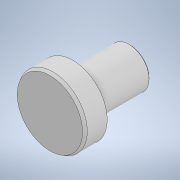
# Autodesk Inventor part: Totmannknopf
Saved by Autodesk Inventor 2021 (Build 250183000, 183)
## iProperties
Created: 2021-07-19
Part Number: Totmannknopf
Material: Generisch
Document SubType Name: Modeling
Designer: Lars-Ole
Density: 1 g/cm^3
Appearance: Vorgabe
Author: Lars-Ole
Autodesk Inventor part; units mm, degrees
ref_plane "YZ Plane" through (0, 0, 0) normal (1, 0, 0) x (0, 1, 0)
ref_plane "XZ Plane" through (0, 0, 0) normal (0, 1, 0) x (-1, 0, 0)
ref_plane "XY Plane" through (0, 0, 0) normal (0, 0, 1) x (1, 0, 0)
sketch "Skizze1" plane through (0, 0, 0) normal (0, 0, 1) x (1, 0, 0)
  line L0 (-2.05, 0.55) -> (2.05, 0.55)
  line L1 (2.05, 0.55) -> (2.05, -0.55)
  line L2 (2.05, -0.55) -> (-2.05, -0.55)
  line L3 (-2.05, -0.55) -> (-2.05, 0.55)
  line L4 (-0.65, 2.05) -> (0.65, 2.05)
  line L5 (0.65, 2.05) -> (0.65, -2.05)
  line L6 (0.65, -2.05) -> (-0.65, -2.05)
  line L7 (-0.65, -2.05) -> (-0.65, 2.05)
  circle A0 centre (0, 0) radius 3.5
  line L8 (-4.9, 0) -> (4.9, 0) construction
  line L9 (0, -4.9) -> (0, 4.9) construction
  point P0 (0.65, -0.55)
  point P1 (-0.65, -0.55)
  point P2 (-0.65, 0.55)
  point P3 (0.65, 0.55)
  dimension "d0" = 1.3
  dimension "d1" = 1.1
  dimension "d2" = 4.1
  dimension "d3" = 4.1
  dimension "d4" = 7
  constraints: 16 end point, 4 parallel, 2 horizontal, 2 perpendicular, 1 centre point, 1 coincident, 4 other
  measures "d0" distance of L4.start L4.end
  measures "d1" distance of L0.end L1.end
  measures "d2" distance between parallel lines of L6 L4
  measures "d3" distance between parallel lines of L3 L1
  measures "d4" diameter of A0
extrude "Extrusion1" add sketch "Skizze1" along normal blind 5
sketch "Skizze2" plane through (0, 0, 5) normal (0, 0, 1) x (1, 0, 0)
  circle A0 centre (0, 0) radius 3.5 projected
extrude "Extrusion2" add sketch "Skizze2" along normal blind 5
sketch "Skizze3" plane through (0, 0, 10) normal (0, 0, 1) x (1, 0, 0)
  circle A0 centre (0, 0) radius 6
  dimension "d9" = 12
  constraints: 1 centre point, 1 coincident
  measures "d9" diameter of A0
extrude "Extrusion3" add sketch "Skizze3" along normal blind 4
chamfer "Fase1" distance 0.3 angle 60 1 edges at (-6, 0, 14) measured on face at (-0.7092, 1.4219, 14)
fillet "Rundung1" radius 0.3 1 edges at (-3.5, 0, 10)
chamfer "Fase2" distance 0.2 angle 45 1 edges at (-3.5, 0, 0)
fillet "Rundung2" radius 0.3 4 edges at (0.65, -0.55, 2.5) (-0.65, -0.55, 2.5) (0.65, 0.55, 2.5) (-0.65, 0.55, 2.5)
